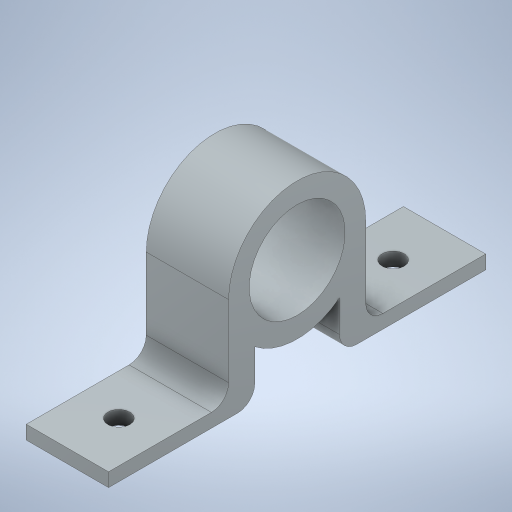
# Autodesk Inventor part: Soporte_cojinete
Saved by Autodesk Inventor 2024 (Build 280153020, 153B)
## iProperties
Created: 2023-05-22
Part Number: Soporte_cojinete
Material: Generic
Document SubType Name: Modeling
Designer: Diego
Density: 1 g/cm^3
Appearance: Default
Author: Diego
Autodesk Inventor part; units mm, degrees
ref_plane "YZ Plane" through (0, 0, 0) normal (1, 0, 0) x (0, 1, 0)
ref_plane "XZ Plane" through (0, 0, 0) normal (0, 1, 0) x (-1, 0, 0)
ref_plane "XY Plane" through (0, 0, 0) normal (0, 0, 1) x (1, 0, 0)
sketch "Sketch1" plane through (0, 0, 0) normal (1, 0, 0) x (0, 1, 0)
  circle A0 centre (0, 0) radius 7
  line L0 (0, 10) -> (-10.5, 10)
  line L1 (0, -10) -> (-10.5, -10)
  line L2 (-7.8658, 6.1749) -> (-12.5, 6.1749)
  line L3 (-15, 8.6749) -> (-15, 15.4804)
  arc A1 (-13, 12.5) -> (-10.5, 10) centre (-10.5, 12.5) ccw
  arc A2 (-15, 8.6749) -> (-12.5, 6.1749) centre (-12.5, 8.6749) ccw
  line L4 (-15, 20.163) -> (-15, 15.4804)
  line L5 (0, 0) -> (-13.6801, 0) construction
  line L6 (-7.8658, -6.1749) -> (-12.5, -6.1749)
  arc A3 (-7.8658, 6.1749) -> (-7.8658, -6.1749) centre (0, 0) ccw
  arc A4 (0, -10) -> (0, 10) centre (0, 0) ccw
  line L7 (-13, 12.5) -> (-13, 27.5)
  line L8 (-13, 27.5) -> (-15, 27.5)
  line L9 (-15, 27.5) -> (-15, 20.163)
  line L10 (-7.8658, -6.1749) -> (-12.5, -6.1749)
  line L11 (-15, -8.6749) -> (-15, -15.4804)
  arc A5 (-10.5, -10) -> (-13, -12.5) centre (-10.5, -12.5) ccw
  arc A6 (-12.5, -6.1749) -> (-15, -8.6749) centre (-12.5, -8.6749) ccw
  line L12 (-15, -20.163) -> (-15, -15.4804)
  line L13 (-13, -12.5) -> (-13, -27.5)
  line L14 (-15, -27.5) -> (-15, -20.163)
  line L15 (-13, -27.5) -> (-15, -27.5)
  point P0 (-13, 10)
  point P1 (-5.25, -10)
  point P2 (-13, -10)
  dimension "d0" = 14
  dimension "d2" = 13
  dimension "d4" = 2.5
  dimension "d7" = 15
  constraints: 32 end point, 12 point on circle, 11 symmetric about line, 7 centre point, 5 horizontal, 4 tangent, 3 perpendicular, 3 point on line, 2 coincident, 1 equal radius, 1 midpoint, 1 parallel, 1 vertical, 2 other
  measures "d0" diameter of A0
  measures "d2" distance of L0.start point (-13, 10)
  measures "d4" radius of A1
  measures "d7" distance of L7.start L7.end
extrude "Extrusion1" add sketch "Sketch1" along normal blind 12
sketch "Sketch2" plane through (0, -13, 27.5) normal (0, 1, 0) x (1, 0, 0)
  line L0 (0, 15) -> (0, 0) construction
  line L1 (0, 15) -> (12, 15) construction
  line L2 (0, 0) -> (12, 15) construction
  line L3 (12, 15) -> (12, 0) construction
  line L4 (0, 15) -> (12, 0) construction
  circle A0 centre (6, 7.5) radius 1.6
  point P0 (0, 27.5)
  dimension "d8" = 3.2
  constraints: 4 end point, 1 centre point, 1 midpoint
  measures "d8" diameter of A0
extrude "Extrusion2" cut sketch "Sketch2" against normal blind 12
sketch "Sketch3" plane through (0, -13, -12.5) normal (0, 1, 0) x (1, 0, 0)
  line L0 (12, -3.8251) -> (12, 15) construction
  line L1 (12, 15) -> (0, 0.0025) construction
  line L2 (0, -3.8251) -> (0, 15) construction
  line L3 (12, 0.0025) -> (0, 15) construction
  circle A0 centre (6, 7.5012) radius 1.6
  point P0 (0, -12.5)
  dimension "d11" = 3.2
  constraints: 4 end point, 1 centre point, 1 midpoint, 1 point on line
  measures "d11" diameter of A0
extrude "Extrusion3" cut sketch "Sketch3" against normal blind 12
body "Solid1"
